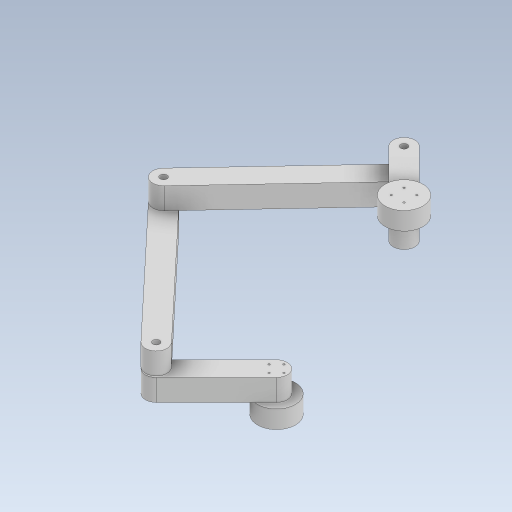
# Autodesk Inventor part: 5 Barras Simplificado
Saved by Autodesk Inventor 2024.2 (Build 282272000, 272)
## iProperties
Created: 2024-02-01
Part Number: 5 Barras Simplificado
Material: Generic
Document SubType Name: Modeling
Designer: juanp
Density: 1 g/cm^3
Appearance: Default
Author: juanp
Autodesk Inventor part; units mm, degrees
ref_plane "YZ Plane" through (0, 0, 0) normal (1, 0, 0) x (0, 1, 0)
ref_plane "XZ Plane" through (0, 0, 0) normal (0, 1, 0) x (-1, 0, 0)
ref_plane "XY Plane" through (0, 0, 0) normal (0, 0, 1) x (1, 0, 0)
sketch "Sketch1" plane through (0, 0, 0) normal (0, 1, 0) x (-1, 0, 0)
  line L0 (1000, 500) -> (0, 500) construction
  line L1 (0, 500) -> (0, -500) construction
  line L2 (0, -500) -> (1000, -500) construction
  line L3 (1000, -500) -> (1000, 500) construction
  line L4 (0, 150) -> (0, -150) construction
  line L5 (25.4, 150) -> (25.4, -150)
  line L6 (-25.4, -150) -> (-25.4, 150)
  arc A0 (25.4, 150) -> (-25.4, 150) centre (0, 150) ccw
  arc A1 (-25.4, -150) -> (25.4, -150) centre (0, -150) ccw
  line L7 (141.4214, 291.4214) -> (0, 150) construction
  line L8 (123.4608, 309.3819) -> (-17.9605, 167.9605)
  line L9 (17.9605, 132.0395) -> (159.3819, 273.4608)
  arc A2 (159.3819, 273.4608) -> (123.4608, 309.3819) centre (141.4214, 291.4214) ccw
  arc A3 (-17.9605, 167.9605) -> (17.9605, 132.0395) centre (0, 150) ccw
  line L10 (141.4214, -291.4214) -> (0, -150) construction
  line L11 (159.3819, -273.4608) -> (17.9605, -132.0395)
  line L12 (-17.9605, -167.9605) -> (123.4608, -309.3819)
  arc A4 (123.4608, -309.3819) -> (159.3819, -273.4608) centre (141.4214, -291.4214) ccw
  arc A5 (17.9605, -132.0395) -> (-17.9605, -167.9605) centre (0, -150) ccw
  line L13 (141.4214, 291.4214) -> (415.417, 0) construction
  line L14 (159.9266, 308.8201) -> (433.9222, 17.3987)
  line L15 (396.9117, -17.3987) -> (122.9161, 274.0226)
  arc A6 (159.9266, 308.8201) -> (122.9161, 274.0226) centre (141.4214, 291.4214) ccw
  arc A7 (396.9117, -17.3987) -> (433.9222, 17.3987) centre (415.417, 0) ccw
  line L16 (141.4214, -291.4214) -> (415.417, 0) construction
  line L17 (159.9266, -308.8201) -> (433.9222, -17.3987)
  line L18 (396.9117, 17.3987) -> (122.9161, -274.0226)
  arc A8 (122.9161, -274.0226) -> (159.9266, -308.8201) centre (141.4214, -291.4214) ccw
  arc A9 (433.9222, -17.3987) -> (396.9117, 17.3987) centre (415.417, 0) ccw
  line L19 (141.4214, -291.4214) -> (141.4214, -558.8873) construction
  line L20 (141.4214, 291.4214) -> (141.4214, 228.8302) construction
  point P0 (0, 0)
  point P1 (0, 0)
  point P2 (0, 0)
  point P3 (70.7107, 220.7107)
  point P4 (70.7107, -220.7107)
  point P5 (278.4192, 145.7107)
  point P6 (278.4192, -145.7107)
  point P7 (-17.9605, 167.9605)
  point P8 (123.4608, -309.3819)
  point P9 (159.9266, -308.8201)
  point P10 (433.9222, -17.3987)
  point P11 (433.9222, 17.3987)
  point P12 (159.9266, 308.8201)
  point P13 (123.4608, 309.3819)
  point P14 (-25.4, -150)
  point P15 (-17.9605, -167.9605)
  dimension "d42" = 1000
  dimension "d43" = 1000
  dimension "d45" = 300
  dimension "d46" = 50.8
  dimension "d47" = 50.8
  dimension "d48" = 50.8
  dimension "d49" = 50.8
  dimension "d50" = 50.8
  dimension "d51" = 200
  dimension "d52" = 200
  dimension "d53" = 400
  dimension "d54" = 400
  dimension "d71" = 136.765
  dimension "d72" = 43.235
  dimension "d73" = 278.4192
  dimension "d74" = 145.7107
  dimension "d75" = 70.7107
  dimension "d76" = 220.7107
  dimension "d77" = 91.765
  dimension "d78" = 150
  dimension "d126" = 45
  dimension "d127" = 45
  constraints: 52 end point, 20 point on circle, 20 tangent, 10 centre point, 7 parallel, 6 midpoint, 3 vertical, 2 coincident, 1 horizontal, 1 perpendicular
  measures "d42" distance of L2.end L1.end
  measures "d43" distance of L2.end L0.start
  measures "d45" distance of L4.start L4.end
  measures "d46" distance between parallel lines of L5 L6
  measures "d47" distance between parallel lines of L14 L15
  measures "d48" distance between parallel lines of L17 L18
  measures "d49" distance between parallel lines of L9 L8
  measures "d50" distance between parallel lines of L12 L11
  measures "d51" distance of L4.start L7.start
  measures "d52" distance of L4.end L10.start
  measures "d53" distance of L13.end L7.start
  measures "d54" distance of L10.start L13.end
  measures "d71" angle of L16 L19
  measures "d72" angle of L13 L20
  measures "d73" distance from line of point (278.419, -145.711) L1
  measures "d74" vertical distance of point (278.419, -145.711) point (0, 0)
  measures "d75" horizontal distance of point (70.711, -220.711) point (0, 0)
  measures "d76" vertical distance of point (70.711, -220.711) point (0, 0)
  measures "d77" angle of L13 L7
  measures "d78" distance of L4.start point (0, 0)
  measures "d126" angle of L10 L4
  measures "d127" angle of L7 L1
extrude "Extrusion6" add sketch "Sketch1" against normal blind 50.8 contours A0 L8 A6 L15 L9 L5 | L5 L9 A3 A0 | L15 A6 A2 L9
extrude "Extrusion7" add sketch "Sketch1" along normal blind 53.8 separate body contours L15 A6 A2 L9 | L9 A2 L14 A9 L18 L15 | L18 A9 A7 L15
extrude "Extrusion13" cut sketch "Sketch1" along normal blind 3 contours L15 A6 A2 L9 | L9 A2 L14 A9 L18 L15 | L18 A9 A7 L15 bodies 2
extrude "Extrusion8" add sketch "Sketch1" along normal blind 107.6 separate body contours L18 L15 A7 L17 A4 L11 | L11 A4 A8 L18 | L18 A9 A7 L15
extrude "Extrusion10" cut sketch "Sketch1" along normal blind 56.8 contours L18 L15 A7 L17 A4 L11 | L11 A4 A8 L18 | L18 A9 A7 L15 bodies 3
extrude "Extrusion9" add sketch "Sketch1" along normal blind 161.4 separate body contours L11 L18 A8 L12 A1 L5 | L5 A1 A5 L11 | L11 A4 A8 L18
extrude "Extrusion11" cut sketch "Sketch1" along normal blind 110.6 contours L11 L18 A8 L12 A1 L5 | L5 A1 A5 L11 | L11 A4 A8 L18 bodies 4
sketch "Sketch6" plane through (0, 0, 0) normal (0, 1, 0) x (1, 0, 0)
  arc A0 (17.9605, -167.9605) -> (-17.9605, -132.0395) centre (0, -150) ccw construction
  line L0 (0, -167.5) -> (-17.5, -150) construction
  line L1 (-17.5, -150) -> (0, -132.5) construction
  line L2 (0, -132.5) -> (17.5, -150) construction
  line L3 (17.5, -150) -> (0, -167.5) construction
  line L4 (0, -167.5) -> (0, -132.5) construction
  line L5 (-17.5, -150) -> (17.5, -150) construction
  circle A1 centre (0, -150) radius 17.5 construction
  line L6 (-123.4608, -309.3819) -> (17.9605, -167.9605) construction
  circle A2 centre (0, -167.5) radius 2.15
  circle A3 centre (-17.5, -150) radius 2.15
  circle A4 centre (17.5, -150) radius 2.15
  circle A5 centre (0, -132.5) radius 2.15
  arc A6 (-159.3819, -273.4608) -> (-123.4608, -309.3819) centre (-141.4214, -291.4214) ccw construction
  circle A7 centre (-141.4214, -291.4214) radius 8.075
  circle A8 centre (-141.4214, -291.4214) radius 7.075
  circle A9 centre (-141.4214, -291.4214) radius 7.875
  arc A10 (-433.9222, 17.3987) -> (-396.9117, -17.3987) centre (-415.417, 0) ccw construction
  arc A11 (-123.4608, 309.3819) -> (-159.3819, 273.4608) centre (-141.4214, 291.4214) ccw construction
  circle A12 centre (-415.417, 0) radius 8.075
  circle A13 centre (-141.4214, 291.4214) radius 8.075
  line L7 (0, 132.5) -> (-17.5, 150) construction
  line L8 (-17.5, 150) -> (0, 167.5) construction
  line L9 (0, 167.5) -> (17.5, 150) construction
  line L10 (17.5, 150) -> (0, 132.5) construction
  line L11 (0, 132.5) -> (0, 167.5) construction
  line L12 (-17.5, 150) -> (17.5, 150) construction
  circle A14 centre (0, 150) radius 17.5 construction
  circle A15 centre (0, 132.5) radius 2.15
  circle A16 centre (-17.5, 150) radius 2.15
  circle A17 centre (17.5, 150) radius 2.15
  circle A18 centre (0, 167.5) radius 2.15
  arc A19 (-17.9605, 132.0395) -> (17.9605, 167.9605) centre (0, 150) ccw construction
  line L13 (-159.3819, 273.4608) -> (-17.9605, 132.0395) construction
  point P0 (0, 0)
  dimension "d83" = 35
  dimension "d107" = 35
  dimension "d84" = 4.3
  dimension "d87" = 16.15
  dimension "d90" = 1
  dimension "d96" = 0.2
  dimension "d108" = 4.3
  constraints: 24 end point, 17 coincident, 13 centre point, 8 equal radius, 6 parallel, 4 perpendicular, 3 midpoint, 2 horizontal alignment, 4 other
  measures "d84" diameter of A3
  measures "d87" diameter of A7
  measures "d90" radial gap between concentric circles of A7 A8
  measures "d96" radial gap between concentric circles of A9 A7
  measures "d108" diameter of A16
extrude "Extrusion19" cut sketch "Sketch6" along normal blind 1000 and the other way blind 1000 contours A2 | A3 | A4 | A5 | A7 | A8 | A9 | A12 | A13 | A15 | A16 | A17 | A18 bodies 1 2 3 4
extrude "Extrusion21" add sketch "Sketch6" against normal blind 45.8 separate body contours A9
extrude "Extrusion22" cut sketch "Sketch6" against normal blind 5 contours A9 bodies 5
ref_plane "Work Plane9" through (0, 55.3, 0) normal (0, 1, 0) x (1, 0, 0)
sketch "Sketch11" plane through (0, 55.3, 0) normal (0, 1, 0) x (1, 0, 0)
  line L0 (0, 0) -> (-361.3999, 0)
  constraints: 2 end point, 1 horizontal
sketch "Sketch12" plane through (0, -50.8, 0) normal (0, 1, 0) x (1, 0, 0)
  circle A0 centre (0, -167.5) radius 2.15 projected
  circle A1 centre (-17.5, -150) radius 2.15 projected
  circle A2 centre (17.5, -150) radius 2.15 projected
  circle A3 centre (0, -132.5) radius 2.15 projected
  arc A4 (17.9605, -167.9605) -> (-17.9605, -132.0395) centre (0, -150) ccw projected
  circle A5 centre (0, -150) radius 44.5
  line L0 (15, -165) -> (-15, -165) construction
  line L1 (-15, -165) -> (-15, -135) construction
  line L2 (-15, -135) -> (15, -135) construction
  line L3 (15, -135) -> (15, -165) construction
  line L4 (15, -165) -> (-15, -135) construction
  line L5 (-15, -165) -> (15, -135) construction
  circle A6 centre (-15, -165) radius 2.15
  circle A7 centre (15, -165) radius 2.15
  circle A8 centre (15, -135) radius 2.15
  circle A9 centre (-15, -135) radius 2.15
  point P0 (0, 0)
  dimension "d113" = 89
  dimension "d114" = 30
  dimension "d115" = 4.3
  constraints: 12 end point, 5 centre point, 5 coincident, 3 equal radius, 2 midpoint, 2 parallel, 2 perpendicular, 1 horizontal
  measures "d113" diameter of A5
  measures "d114" distance of L0.end L1.end
  measures "d115" diameter of A6
extrude "Extrusion23" add sketch "Sketch12" against normal blind 42 separate body contours A0 | A1 | A2 | A3 | A5
pattern_circular "Circular Pattern3" count 2 over 360 about axis through (0, 55.3, 0) along (-1, 0, 0) of "Extrusion23" bodies 6
equation "\"d45\" = L_G"
equation "\"d46\" = t"
equation "\"d47\" = t"
equation "\"d48\" = t"
equation "\"d49\" = t"
equation "\"d50\" = t"
equation "\"d51\" = L_P"
equation "\"d52\" = L_P"
equation "\"d53\" = L_D"
equation "\"d54\" = L_D"
equation "\"d57\" = t"
equation "\"d59\" = t + sep"
equation "\"d79\" = sep"
equation "\"d61\" = 2 * t + 2 * sep"
equation "\"L_G\" = 300"
equation "\"L_P\" = 200"
equation "\"L_D\" = 400"
equation "\"t\" = 50.8 * scale"
equation "\"sep\" = 3"
equation "\"scale\" = 1"
body "Solid6"
body "Solid7"
body "Solid8"
body "Solid9"
body "Solid13"
body "Solid14"
